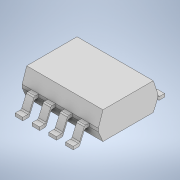
# Autodesk Inventor part: as5600
Saved by Autodesk Inventor 2020 (Build 240168000, 168)
## iProperties
Created: 2019-05-15
Part Number: as5600
Material: Generic
Document SubType Name: Modeling
Designer: psrob
Density: 1 g/cm^3
Appearance: Default
Author: psrob
Autodesk Inventor part; units mm, degrees
ref_plane "YZ Plane" through (0, 0, 0) normal (1, 0, 0) x (0, 1, 0)
ref_plane "XZ Plane" through (0, 0, 0) normal (0, 1, 0) x (-1, 0, 0)
ref_plane "XY Plane" through (0, 0, 0) normal (0, 0, 1) x (1, 0, 0)
sketch "Sketch1" plane through (0, 0, 0) normal (0, 1, 0) x (-1, 0, 0)
  line L0 (2.5, 1.95) -> (2.5, -1.95)
  line L1 (2.5, -1.95) -> (-2.5, -1.95)
  line L2 (-2.5, -1.95) -> (-2.5, 1.95)
  line L3 (-2.5, 1.95) -> (2.5, 1.95)
  line L4 (2.5, 1.95) -> (-2.5, -1.95) construction
  line L5 (2.5, -1.95) -> (-2.5, 1.95) construction
  point P0 (0, 0)
  dimension "d0" = 3.9
  dimension "d1" = 5
  constraints: 12 end point, 2 midpoint, 2 parallel, 1 perpendicular, 1 vertical
  measures "d0" distance of L0.start L0.end
  measures "d1" distance of L2.end L0.start
extrude "Extrusion1" add sketch "Sketch1" along normal blind 1.8
sketch "Sketch2" plane through (2.5, 0, 1.95) normal (1, 0, 0) x (0, 0, -1)
  line L0 (0, 0) -> (3.9, 0) projected
  line L1 (3.9, 0) -> (3.9, 1.8) projected
  line L2 (0, 1.8) -> (3.9, 1.8) projected
  line L3 (0, 0) -> (0, 1.8) projected
  line L4 (0, 0) -> (0, 1.8) projected
  line L5 (0, 0.9) -> (3.9, 0.9)
  line L6 (3.9, 0) -> (3.9, 1.8) projected
  line L7 (0, 0.9) -> (-1.05, 0.9)
  line L8 (3.9, 0.9) -> (4.95, 0.9)
  line L9 (-1.05, 0.9) -> (-1.05, -0.1)
  line L10 (4.95, 0.9) -> (4.95, -0.1)
  line L11 (-1.05, -0.1) -> (-0.65, -0.1)
  line L12 (-0.65, -0.1) -> (-0.65, 0.1)
  line L13 (-0.65, 0.1) -> (-1.05, 0.1)
  line L14 (-1.05, 0.1) -> (-1.05, -0.1)
  line L15 (4.95, -0.1) -> (4.55, -0.1)
  line L16 (4.55, -0.1) -> (4.55, 0.1)
  line L17 (4.55, 0.1) -> (4.95, 0.1)
  line L18 (4.95, 0.1) -> (4.95, -0.1)
  line L19 (0, 0.9) -> (-0.3, 0.9)
  line L20 (-0.3, 0.9) -> (-0.3, 0.7)
  line L21 (-0.3, 0.7) -> (0, 0.7)
  line L22 (0, 0.7) -> (0, 0.9)
  line L23 (3.9, 0.9) -> (4.2, 0.9)
  line L24 (4.2, 0.9) -> (4.2, 0.7)
  line L25 (4.2, 0.7) -> (3.9, 0.7)
  line L26 (3.9, 0.7) -> (3.9, 0.9)
  line L27 (-0.65, 0.1) -> (-0.3, 0.9)
  line L28 (-0.3, 0.7) -> (-0.65, -0.1)
  line L29 (4.2, 0.9) -> (4.55, 0.1)
  line L30 (4.2, 0.7) -> (4.55, -0.1)
  point P0 (1.95, 0)
  dimension "d4" = 1.05
  dimension "d5" = 1.05
  dimension "d6" = 1
  dimension "d7" = 1
  dimension "d8" = 0.4
  dimension "d9" = 0.2
  dimension "d10" = 0.4
  dimension "d11" = 0.2
  dimension "d12" = 0.3
  dimension "d13" = 0.2
  dimension "d14" = 0.3
  dimension "d15" = 0.2
  constraints: 50 end point, 8 parallel, 6 horizontal, 4 perpendicular, 2 midpoint, 2 vertical
  measures "d4" distance of L5.start L7.end
  measures "d5" distance of L5.end L8.end
  measures "d6" distance of L7.end L9.end
  measures "d7" distance of L8.end L10.end
  measures "d8" distance of L13.end L12.end
  measures "d9" distance of L12.end L11.end
  measures "d10" distance of L16.end L17.end
  measures "d11" distance of L15.end L16.end
  measures "d12" distance of L21.end L20.end
  measures "d13" distance of L20.end L19.end
  measures "d14" distance of L24.end L25.end
  measures "d15" distance of L23.end L24.end
sketch "Sketch3" plane through (2.5, 0, 1.95) normal (1, 0, 0) x (0, 0, -1)
  line L0 (0, 1.8) -> (3.9, 1.8) projected
  line L1 (0, 1.8) -> (0.3, 1.8)
  line L2 (0.3, 1.8) -> (0, 0.9)
  line L3 (0, 0) -> (0, 1.8) projected
  line L4 (3.9, 0) -> (3.9, 1.8) projected
  line L5 (3.9, 1.8) -> (3.6, 1.8)
  line L6 (3.6, 1.8) -> (3.9, 0.9)
  line L7 (0, 0) -> (0.3, 0)
  line L8 (0, 0) -> (3.9, 0) projected
  line L9 (0.3, 0) -> (0, 0.6871)
  line L10 (3.9, 0) -> (3.6, 0)
  line L11 (3.6, 0) -> (3.9, 0.6871)
  point P0 (1.95, 0)
  dimension "d16" = 0.3
  dimension "d17" = 0.3
  dimension "d18" = 0.3
  dimension "d19" = 0.3
  constraints: 16 end point, 6 point on line, 1 midpoint
  measures "d16" distance of L0.start L1.end
  measures "d17" distance of L0.end L5.end
  measures "d18" distance of L3.start L7.end
  measures "d19" distance of L4.start L10.end
extrude "Extrusion2" cut sketch "Sketch3" against normal blind 10 contours L0 L2 L3 | L0 L4 L6 | L9 L7 L3 | L4 L8 L11
ref_plane "Work Plane1" through (1.9, 0, 1.65) normal (1, 0, 0) x (0, 0, -1)
sketch "Sketch4" plane through (1.9, 0, 1.65) normal (1, 0, 0) x (0, 0, -1)
  line L0 (3.9, 0.9) -> (3.9, 0.7) projected
  line L1 (3.9, 0.7) -> (3.6, 0.7) projected
  line L2 (3.6, 0.9) -> (4.65, 0.9) projected
  line L3 (3.9, 0.9) -> (4.25, 0.1) projected
  line L4 (3.9, 0.7) -> (4.25, -0.1) projected
  line L5 (4.25, 0.1) -> (4.65, 0.1) projected
  line L6 (4.25, -0.1) -> (4.25, 0.1) projected
  line L7 (4.65, -0.1) -> (4.25, -0.1) projected
  line L8 (4.65, 0.1) -> (4.65, -0.1) projected
  line L9 (-0.95, 0.1) -> (-1.35, 0.1) projected
  line L10 (-1.35, -0.1) -> (-0.95, -0.1) projected
  line L11 (-1.35, 0.9) -> (-1.35, -0.1) projected
  line L12 (-0.6, 0.7) -> (-0.95, -0.1) projected
  line L13 (-0.95, 0.1) -> (-0.6, 0.9) projected
  line L14 (-0.6, 0.9) -> (-0.6, 0.7) projected
  line L15 (-0.95, -0.1) -> (-0.95, 0.1) projected
  line L16 (-0.6, 0.7) -> (-0.3, 0.7) projected
  line L17 (-0.3, 0.6871) -> (-0.3, 0.9) projected
  line L18 (-0.3, 0.9) -> (-0.6, 0.9) projected
  line L19 (-0.3, 0.9) -> (-1.35, 0.9) projected
  line L20 (4.65, 0.9) -> (4.65, -0.1) projected
  line L21 (3.6, 0.7) -> (3.6, 0.9)
  line L22 (0, 1.8) -> (-0.3, 0.9) projected
  line L23 (-0.3, 0.6871) -> (0, 0) projected
  line L24 (-0.3, 0.9) -> (-0.3, 0.6871)
  point P0 (1.65, 0)
  constraints: 4 end point, 1 parallel, 1 vertical
extrude "Extrusion3" add sketch "Sketch4" against normal blind 0.5 contours L3 L6 L4 L0 | L0 L1 L21 L2 | L5 L8 L7 L6 | L15 L10 L11 L9 | L13 L14 L12 L15 | L18 L17 L16 L14
fillet "Fillet1" radius 0.1 8 edges at (1.65, 0.9, -2.25) (1.65, 0.7, -2.25) (1.65, -0.1, -2.6) (1.65, 0.1, -2.6) (1.65, 0.9, 2.25) (1.65, 0.1, 2.6) (1.65, -0.1, 2.6) (1.65, 0.7, 2.25)
pattern_linear "Rectangular Pattern1" count 4 spacing 1.1 along (-1, 0, 0) of "Extrusion3", "Fillet1"
sketch "Sketch5" plane through (1.9, 0, 1.65) normal (1, 0, 0) x (0, 0, -1)
  point P0 (1.65, 0)
body "Solid1"
